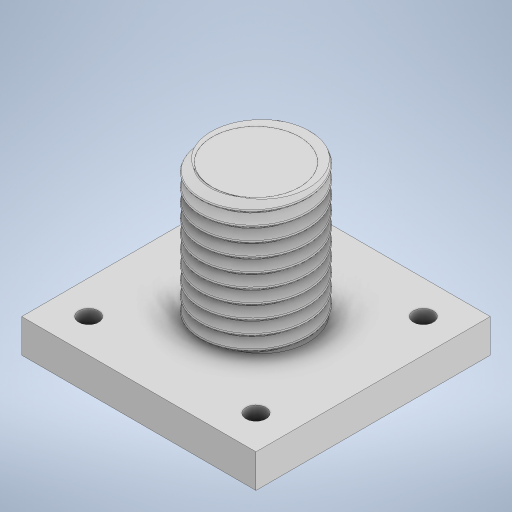
# Autodesk Inventor part: bottom-adaptor
Saved by Autodesk Inventor 2024 (Build 280153000, 153)
## iProperties
Created: 2023-10-19
Part Number: bottom-adaptor
Material: 일반
Document SubType Name: Modeling
Designer: jsw
Density: 1 g/cm^3
Appearance: 기본값
Author: jsw
Autodesk Inventor part; units mm, degrees
ref_plane "YZ Plane" through (0, 0, 0) normal (1, 0, 0) x (0, 1, 0)
ref_plane "XZ Plane" through (0, 0, 0) normal (0, 1, 0) x (-1, 0, 0)
ref_plane "XY Plane" through (0, 0, 0) normal (0, 0, 1) x (1, 0, 0)
sketch "스케치1" plane through (0, 0, 0) normal (0, 1, 0) x (-1, 0, 0)
  line L0 (-17.5, -17.5) -> (17.5, -17.5)
  line L1 (17.5, -17.5) -> (17.5, 17.5)
  line L2 (17.5, 17.5) -> (-17.5, 17.5)
  line L3 (-17.5, 17.5) -> (-17.5, -17.5)
  line L4 (-17.5, -17.5) -> (17.5, 17.5) construction
  line L5 (17.5, -17.5) -> (-17.5, 17.5) construction
  circle A0 centre (12.5, 12.5) radius 1.5
  circle A1 centre (12.5, -12.5) radius 1.5
  circle A2 centre (-12.5, 12.5) radius 1.5
  circle A3 centre (-12.5, -12.5) radius 1.5
  point P0 (0, 0)
  dimension "d0" = 35
  dimension "d1" = 35
  dimension "d2" = 12.5
  dimension "d3" = 3
  dimension "d6" = 25
  dimension "d9" = 25
  constraints: 12 end point, 4 centre point, 2 horizontal, 2 midpoint, 2 parallel, 1 perpendicular, 1 point on line, 1 vertical, 6 other
  measures "d0" distance of L2.end L1.end
  measures "d1" distance of L1.end L0.end
  measures "d2" horizontal distance of point (0, 0) A0.centre
  measures "d3" diameter of A0
  measures "d6" distance of A0.centre A1.centre
  measures "d9" distance of A0.centre A2.centre
extrude "돌출1" add sketch "스케치1" along normal blind 5
sketch "스케치2" plane through (0, 5, 0) normal (0, 1, 0) x (1, 0, 0)
  circle A0 centre (0, 0) radius 8
  dimension "d14" = 16
  constraints: 1 centre point, 1 coincident
  measures "d14" diameter of A0
extrude "돌출2" add sketch "스케치2" along normal blind 20
thread "스레드1" size "M16x2" class "6g" standard "ANSI Metric M Profile" full length
sketch "스케치4" plane through (0, 25, 0) normal (1, 0, 0) x (0, 0, 1)
  line L0 (8, 0) -> (8, 20)
  line L1 (8, 20) -> (6.5171, 20)
  line L2 (6.5171, 20) -> (6.5171, 0)
  line L3 (6.5171, 0) -> (8, 0)
  line L4 (0, -7.6171) -> (0, 30.4362) projected
  constraints: 8 end point
revolve "회전1" cut sketch "스케치4" angle 360 about axis through (0, 25, 0) along (0, -1, 0)
sketch "스케치5" plane through (0, 25, 0) normal (1, 0, 0) x (0, 0, 1)
  line L0 (8, 0) -> (8, 20)
  line L1 (8, 20) -> (6.5171, 20)
  line L2 (6.5171, 20) -> (6.5171, 0)
  line L3 (6.5171, 0) -> (8, 0)
  line L4 (0, -7.6171) -> (0, 30.4362) projected
  constraints: 8 end point
revolve "회전2" add sketch "스케치5" angle 360 about axis through (0, 25, 0) along (0, -1, 0) separate body
sketch "스케치3" plane through (0, 25, 0) normal (-1, 0, 0) x (0, -1, 0)
  line L0 (-1.1668, -6.6184) -> (-1.0001, -6.6184) construction
  line L1 (0.1666, -7.899) -> (-0.0001, -8.2192) construction
  line L2 (-2.0001, -8.2192) -> (-2.1668, -7.899) construction
  line L3 (-0.8334, -6.6184) -> (-1.0001, -6.2982) construction
  line L4 (-1.0001, -6.2982) -> (-1.1668, -6.6184) construction
  line L5 (-2.0001, -8.2192) -> (-1.8334, -7.899) construction
  line L6 (-0.8334, -6.6184) -> (-0.1668, -7.899)
  line L7 (-2.1668, -7.899) -> (-1.8334, -7.899) construction
  arc A0 (-2.1668, -7.899) -> (-2.0001, -8.0002) centre (-2.0001, -7.8123) ccw construction
  line L8 (0.1666, -7.899) -> (-0.1668, -7.899) construction
  line L9 (-2.0001, -8.2192) -> (-2.0001, -7.899) construction
  line L10 (-0.0001, -8.2192) -> (-0.0001, -7.899) construction
  line L11 (-1.0001, -6.2982) -> (-1.0001, -6.5172) construction
  line L12 (-2.0001, -8.0002) -> (-0.0001, -8.0002)
  arc A1 (-2.0001, -8.0002) -> (-1.8334, -7.899) centre (-2.0001, -7.8123) ccw
  line L13 (-0.1668, -7.899) -> (-0.0001, -8.2192) construction
  line L14 (-1.8334, -7.899) -> (-1.1668, -6.6184)
  line L15 (-0.0001, -0.0002) -> (-0.0001, 0.0177)
  line L16 (-0.0001, 0.0177) -> (-0.0001, -0.0002)
  line L17 (-0.0001, -0.0002) -> (0.0334, -0.0002)
  arc A2 (-0.1668, -7.899) -> (-0.0001, -8.0002) centre (-0.0001, -7.8123) ccw
  arc A3 (-0.0001, -8.0002) -> (0.1666, -7.899) centre (-0.0001, -7.8123) ccw construction
  arc A4 (-1.0001, -6.5172) -> (-1.1668, -6.6184) centre (-1.0001, -6.7051) ccw
  arc A5 (-0.8334, -6.6184) -> (-1.0001, -6.5172) centre (-1.0001, -6.7051) ccw
  line L18 (-1.0001, -6.5172) -> (-1.0001, -6.6184) construction
  line L19 (-1.0001, -6.6184) -> (-0.8334, -6.6184) construction
  dimension "d19" = 55
  dimension "d20" = 0.3202
  dimension "d21" = 0.3202
  dimension "d24" = 2
  constraints: 40 end point, 12 point on circle, 10 parallel, 8 tangent, 7 collinear, 6 centre point, 2 midpoint, 2 point on line, 1 horizontal, 1 perpendicular, 5 other
  measures "d19" angle of L6 L14
  measures "d20" distance of L3.end L0.end
  measures "d21" distance of L1.end L10.end
  measures "d24" distance from line of L1.end L9
coil "코일1" sketch "스케치3" operation cut axis through (0, 25, 0) along (0, -1, 0) pitch 2.002 turns 11.988012 hand right bodies 2
equation "\"d19\" = d26"
equation "\"d26\" = 55deg"
